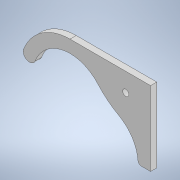
# Autodesk Inventor part: FlexiHook
Saved by Autodesk Inventor 2022 (Build 260153000, 153)
## iProperties
Created: 2022-03-07
Part Number: FlexiHook
Material: Generic
Document SubType Name: Modeling
Designer: tagaz
Density: 1 g/cm^3
Appearance: Default
Author: tagaz
Autodesk Inventor part; units mm, degrees
ref_plane "YZ Plane" through (0, 0, 0) normal (1, 0, 0) x (0, 1, 0)
ref_plane "XZ Plane" through (0, 0, 0) normal (0, 1, 0) x (-1, 0, 0)
ref_plane "XY Plane" through (0, 0, 0) normal (0, 0, 1) x (1, 0, 0)
sketch "Sketch1" plane through (0, 0, 0) normal (0, 0, 1) x (1, 0, 0)
  line L0 (0, 0) -> (50.8, 0)
  line L1 (50.8, 0) -> (50.8, 76.2)
  line L2 (50.8, 76.2) -> (0, 76.2)
  line L3 (0, 38.1) -> (0, 0)
  line L4 (0, 76.2) -> (-63.5, 76.2)
  arc A0 (1.7585, 54.6059) -> (-73.2671, 41.2788) centre (-31.75, 25.4) ccw construction
  arc A1 (0.97, 64.2593) -> (-79.1981, 43.5472) centre (-31.75, 25.4) ccw
  arc A2 (-3.0285, 50.4336) -> (-67.336, 39.0104) centre (-31.75, 25.4) ccw
  arc A3 (-3.0285, 50.4336) -> (-4.2902, 56.5386) centre (1.7585, 54.6059) ccw
  arc A4 (-79.1981, 43.5472) -> (-67.336, 39.0104) centre (-73.2671, 41.2788) ccw
  line L5 (-3.0285, 50.4336) -> (0, 38.1)
  point P0 (-31.75, 76.2)
  dimension "d7" = 50.8
  dimension "d8" = 76.2
  dimension "d11" = 50.8
  dimension "d33" = 38.1
  dimension "d34" = 63.5
  dimension "d35" = 76.2
  dimension "d36" = 44.45
  dimension "d37" = 12.7
  dimension "d38" = 38.1
  dimension "d39" = 31.75
  dimension "d42" = 12.7
  constraints: 12 end point, 10 point on circle, 5 centre point, 5 tangent, 2 horizontal, 2 parallel, 1 coincident, 1 perpendicular, 1 other
  measures "d7" distance of L2.end L1.end
  measures "d8" distance of L1.end L0.end
  measures "d11" distance of L0.start L0.end
  measures "d33" distance of L3.start L0.start
  measures "d34" distance of L2.end L4.end
  measures "d35" distance of A0.end A0.start
  measures "d36" radius of A0
  measures "d37" diameter of A3
  measures "d38" radius of A2
  measures "d39" distance from line of L3 A0.centre
  measures "d42" distance of L5.start L3.start
extrude "Extrusion1" add sketch "Sketch1" along normal blind 6.35
sketch "Sketch2" plane through (0, 0, 6.35) normal (0, 0, 1) x (1, 0, 0)
  line L0 (0, 0) -> (50.8, 0) projected
  circle A0 centre (0, 0) radius 38.1
  dimension "d16" = 76.2
  constraints: 1 centre point
  measures "d16" diameter of A0
extrude "Extrusion2" cut sketch "Sketch2" against normal blind 6.35
fillet "Fillet1" radius 3.175 1 edges at (38.1, 0, 3.175)
sketch "Sketch3" plane through (0, 0, 6.35) normal (0, 0, 1) x (1, 0, 0)
  circle A0 centre (25.4, 57.15) radius 3.175
  line L0 (50.8, 76.2) -> (-31.75, 76.2) projected
  line L1 (41.1527, 0) -> (50.8, 0) projected
  point P0 (0, 0)
  point P1 (25.4, 76.2)
  point P2 (0, 76.2)
  dimension "d20" = 6.35
  dimension "d22" = 19.05
  constraints: 1 centre point, 1 point on line, 1 vertical alignment
  measures "d20" diameter of A0
  measures "d22" distance from line of L0 A0.centre
extrude "Extrusion3" cut sketch "Sketch3" against normal blind 6.35
sketch "Sketch4" plane through (0, 0, 6.35) normal (0, 0, 1) x (1, 0, 0)
  circle A0 centre (32.5341, 12.7) radius 3.175 construction
  line L0 (50.8, 76.2) -> (-31.75, 76.2) construction
  arc A1 (37.9871, 2.9308) -> (0, 38.1) centre (0, 0) ccw construction
  point P0 (0, 76.2)
  point P1 (25.4, 76.2)
  point P2 (2.9308, 37.9871)
  point P3 (-3.3199, 37.9551)
  dimension "d25" = 6.35
  dimension "d26" = 63.5
  constraints: 1 centre point, 1 point on line, 1 tangent
  measures "d25" diameter of A0
  measures "d26" distance from line of L0 A0.centre
fillet "Fillet2" radius 82.55 1 edges at (0, 38.1, 3.175)
body "Solid358"
